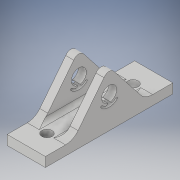
# Autodesk Inventor part: TestingBracket
Saved by Autodesk Inventor 2018 (Build 220112000, 112)
## iProperties
Created: 2019-06-20
Part Number: TestingBracket
Material: Generic
Document SubType Name: Modeling
Designer: anirudh
Density: 1 g/cm^3
Appearance: Default
Author: anirudh
Autodesk Inventor part; units mm, degrees
ref_plane "YZ Plane" through (0, 0, 0) normal (1, 0, 0) x (0, 1, 0)
ref_plane "XZ Plane" through (0, 0, 0) normal (0, 1, 0) x (-1, 0, 0)
sketch "Sketch1" plane through (0, 0, 0) normal (0, 1, 0) x (-1, 0, 0)
  line L0 (0, 0) -> (30.48, 0)
  line L1 (30.48, 0) -> (30.48, -101.6)
  line L2 (30.48, -101.6) -> (0, -101.6)
  line L3 (0, -101.6) -> (0, 0)
  circle A0 centre (15.24, -16.51) radius 4.1275
  circle A1 centre (15.24, -85.09) radius 4.1275
  dimension "d0" = 30.48
  dimension "d1" = 101.6
  dimension "d4" = 8.255
  dimension "d5" = 8.255
  constraints: 8 end point, 2 centre point, 2 parallel, 1 horizontal, 1 perpendicular
  measures "d0" distance of L1.end L2.end
  measures "d1" distance of L0.end L1.end
  measures "d4" diameter of A0
  measures "d5" diameter of A1
extrude "Extrusion1" add sketch "Sketch1" along normal blind 7.62
sketch "Sketch2" plane through (0, 0, 0) normal (1, 0, 0) x (0, 0, -1)
  line L0 (0, 0) -> (0, 7.62) projected
  line L1 (0, 7.62) -> (101.6, 7.62) projected
  line L2 (0, 7.62) -> (101.6, 7.62)
  arc A0 (51.8409, 19.4967) -> (49.7591, 19.4967) centre (50.8, 25.4) ccw
  arc A1 (44.3162, 18.9162) -> (57.2837, 18.9163) centre (50.8, 25.4) ccw
  line L3 (50.8, 25.4) -> (59.9694, 25.4) construction
  line L4 (50.8, 25.4) -> (59.9694, 25.4) construction
  arc A2 (45.4388, 20.0388) -> (44.3162, 18.9162) centre (44.8775, 19.4775) ccw
  arc A3 (57.2837, 18.9163) -> (56.1612, 20.0388) centre (56.7225, 19.4775) ccw
  line L5 (50.8, 25.4) -> (58.3819, 25.4) construction
  arc A4 (48.1597, 18.2927) -> (49.7591, 19.4967) centre (48.3236, 19.7391) ccw
  arc A5 (51.8409, 19.4967) -> (53.4403, 18.2927) centre (53.2763, 19.7391) ccw
  arc A6 (45.4388, 20.0388) -> (48.1597, 18.2927) centre (50.8, 25.4) ccw
  arc A7 (53.4403, 18.2927) -> (56.1612, 20.0388) centre (50.8, 25.4) ccw
  line L6 (50.8, 7.62) -> (22.225, 7.62)
  arc A8 (54.8949, 38.7005) -> (46.7051, 38.7005) centre (50.8, 36.195) ccw
  line L7 (22.225, 7.62) -> (46.7051, 38.7005)
  line L8 (50.8, 7.62) -> (79.375, 7.62)
  line L9 (79.375, 7.62) -> (54.8949, 38.7005)
  dimension "d16" = 28.575
  dimension "d17" = 28.575
  constraints: 22 point on circle, 16 end point, 9 centre point, 3 horizontal, 2 coincident, 2 point on line, 1 collinear, 1 midpoint, 1 tangent
  measures "d16" distance of L6.start L6.end
  measures "d17" distance of L6.start L8.end
extrude "Extrusion2" add sketch "Sketch2" against normal blind 6.35
ref_plane "Work Plane1" through (-15.24, 0, -101.6) normal (-1, 0, 0) x (0, 0, 1)
mirror "Mirror1" about plane through (-15.24, 0, -101.6) normal (-1, 0, 0) of "Extrusion2"
fillet "Fillet1" radius 12.7 4 edges at (-3.175, 7.62, -79.375) (-27.305, 7.62, -79.375) (-27.305, 7.62, -22.225) (-3.175, 7.62, -22.225)
fillet "Fillet3" radius 3.175 2 edges at (-24.13, 7.62, -50.8) (-6.35, 7.62, -50.8)
body "Solid1"
